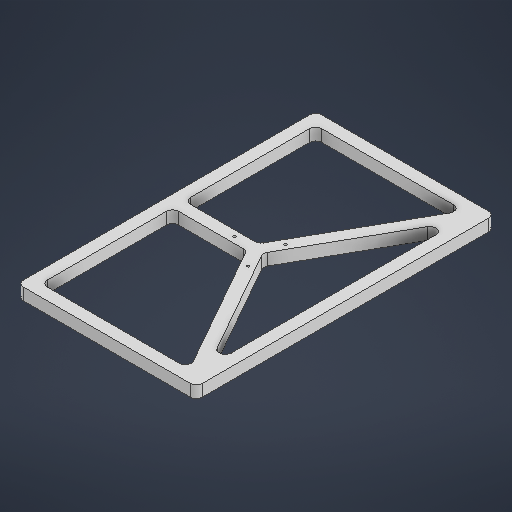
# Autodesk Inventor part: Aufhängung
Saved by Autodesk Inventor 2027 (Build 310192060, 192F)
## iProperties
Created: 2016-02-20
Part Number: Aufhängung
Material: Generisch
Document SubType Name: Modeling
Designer: Halle20
Density: 1 g/cm^3
Appearance: Vorgabe
Author: Halle20
Autodesk Inventor part; units mm, degrees
ref_plane "YZ Plane" through (0, 0, 0) normal (1, 0, 0) x (0, 1, 0)
ref_plane "XZ Plane" through (0, 0, 0) normal (0, 1, 0) x (-1, 0, 0)
ref_plane "XY Plane" through (0, 0, 0) normal (0, 0, 1) x (1, 0, 0)
sketch "Sketch5" plane through (0, 0, 0) normal (0, 0, 1) x (1, 0, 0)
  line L0 (0, 0) -> (300, 0)
  line L1 (300, 0) -> (300, 500)
  line L2 (300, 500) -> (0, 500)
  line L3 (0, 500) -> (0, 0)
  line L4 (20, 480) -> (280, 480)
  line L5 (280, 480) -> (280, 20)
  line L6 (280, 20) -> (20, 20)
  line L7 (20, 20) -> (20, 480)
  line L8 (150, 0) -> (150, 500)
  circle A0 centre (150, 250) radius 36
  circle A1 centre (114, 250) radius 2
  circle A2 centre (168, 218.8231) radius 2
  circle A3 centre (168, 281.1769) radius 2
  line L9 (20, 250) -> (150, 250)
  line L10 (20, 240) -> (150, 240)
  line L11 (20, 260) -> (150, 260)
  line L12 (280, 20) -> (150, 250)
  line L13 (150, 250) -> (280, 480)
  line L14 (271.2944, 15.0794) -> (141.2944, 245.0794)
  line L15 (288.7056, 24.9206) -> (158.7056, 254.9206)
  line L16 (158.7056, 245.0794) -> (288.7056, 475.0794)
  line L17 (141.2944, 254.9206) -> (271.2944, 484.9206)
  point P0 (161.4868, 250)
  point P1 (280, 459.6772)
  point P2 (280, 40.3228)
  point P3 (144.1654, 240)
  point P4 (268.5132, 20)
  point P5 (268.5132, 480)
  point P6 (144.1654, 260)
  dimension "d31" = 72
  dimension "d28" = 300
  dimension "d29" = 500
  dimension "d30" = 20
  dimension "d32" = 4
  dimension "d35" = 360
  dimension "d37" = 10
  dimension "d38" = 10
  dimension "d39" = 10
  dimension "d40" = 10
  dimension "d41" = 10
  dimension "d42" = 10
  constraints: 36 end point, 10 parallel, 4 midpoint, 3 centre point, 3 perpendicular, 1 horizontal, 1 horizontal alignment, 12 other
  measures "d28" distance of L2.end L1.end
  measures "d29" distance of L1.end L0.end
  measures "d30" distance between parallel lines of L2 L4
  measures "d32" diameter of A1
  measures "d37" distance between parallel lines of L9 L10
  measures "d38" distance between parallel lines of L9 L11
  measures "d39" distance between parallel lines of L12 L14
  measures "d40" distance between parallel lines of L12 L15
  measures "d41" distance between parallel lines of L13 L16
  measures "d42" distance between parallel lines of L13 L17
extrude "Extrusion5" add sketch "Sketch5" along normal blind 20 contours L3 L2 L8 L4 L7 L6 L0 | L8 L6 L5 L4 L2 L1 L0 | L14 A0 A2 L12 L6 | L12 A2 A0 L15 L5 | L14 L8 L12 A2 A0 | L7 L9 A1 A0 L10 | L14 L10 L8 | A0 A1 L9 L8 L10 | L4 L13 A3 A0 L17 | L12 A0 A2 | A2 A0 L12 | A2 L12 A0 | L7 L11 A0 A1 L9 | A1 L9 A0 | A0 L9 A1 | L5 L16 A0 A3 L13 | A0 A3 L13 L8 L17 | L8 L11 L17 | L11 L8 L9 A1 A0 | A0 A2 L12 L13 A3 L16 L15 | L12 A2 A0 | A1 A0 L9 | A0 A1 L9 | L13 A0 A3 | A3 A0 L13 | A0 L13 A3 | L13 A0 A3
hole "Hole1" at (168, 218.8231, 0) at (168, 281.1769, 0) at (114, 250, 0) direction (0, 0, 1) diameter 4.3 depth 20 clearance for "Socket Head Cap Screw ISO 4762" size "M4" standard "ISO"
fillet "Fillet1" radius 10 15 edges at (0, 0, 10) (20, 20, 10) (300, 0, 10) (268.5132, 20, 10) (280, 40.3228, 10) (144.1654, 240, 10) (144.1654, 260, 10) (161.4868, 250, 10) (20, 240, 10) (20, 260, 10) (0, 500, 10) (20, 480, 10) (300, 500, 10) (268.5132, 480, 10) (280, 459.6772, 10)
body "Solid3"
